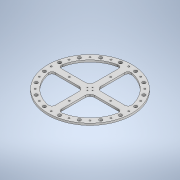
# Autodesk Inventor part: 24_Disco
Saved by Autodesk Inventor 2020.2 (Build 242310000, 310)
## iProperties
Created: 2019-11-29
Part Number: 24_Disco
Material: Generico
Document SubType Name: Modeling
Designer: socci
Density: 1 g/cm^3
Appearance: Default
Author: socci
Autodesk Inventor part; units mm, degrees
ref_plane "YZ Plane" through (0, 0, 0) normal (1, 0, 0) x (0, 1, 0)
ref_plane "XZ Plane" through (0, 0, 0) normal (0, 1, 0) x (-1, 0, 0)
ref_plane "XY Plane" through (0, 0, 0) normal (0, 0, 1) x (1, 0, 0)
sketch "Schizzo1" plane through (0, 0, 0) normal (0, 1, 0) x (-1, 0, 0)
  circle A0 centre (0, 0) radius 130
  line L0 (0, 130) -> (0, -130)
  line L1 (130, 0) -> (-130, 0)
  line L2 (10, 97.9796) -> (10, 23.6854)
  line L3 (97.9796, 10) -> (23.6854, 10)
  arc A1 (16.045, 13.5484) -> (13.5484, 16.045) centre (0, 0) ccw
  arc A2 (107.7775, 22) -> (22, 107.7775) centre (0, 0) ccw
  arc A3 (22, 107.7775) -> (10, 97.9796) centre (20, 97.9796) ccw
  arc A4 (10, 23.6854) -> (13.5484, 16.045) centre (20, 23.6854) ccw
  arc A5 (16.045, 13.5484) -> (23.6854, 10) centre (23.6854, 20) ccw
  arc A6 (97.9796, 10) -> (107.7775, 22) centre (97.9796, 20) ccw
  arc A7 (-13.5484, 16.045) -> (-10, 23.6854) centre (-20, 23.6854) ccw
  arc A8 (-13.5484, 16.045) -> (-16.045, 13.5484) centre (0, 0) ccw
  arc A9 (-23.6854, 10) -> (-16.045, 13.5484) centre (-23.6854, 20) ccw
  line L4 (-10, 97.9796) -> (-10, 23.6854)
  line L5 (-97.9796, 10) -> (-23.6854, 10)
  arc A10 (-107.7775, 22) -> (-97.9796, 10) centre (-97.9796, 20) ccw
  arc A11 (-22, 107.7775) -> (-107.7775, 22) centre (0, 0) ccw
  arc A12 (-10, 97.9796) -> (-22, 107.7775) centre (-20, 97.9796) ccw
  arc A13 (-16.045, -13.5484) -> (-23.6854, -10) centre (-23.6854, -20) ccw
  arc A14 (-16.045, -13.5484) -> (-13.5484, -16.045) centre (0, 0) ccw
  arc A15 (-10, -23.6854) -> (-13.5484, -16.045) centre (-20, -23.6854) ccw
  line L6 (-97.9796, -10) -> (-23.6854, -10)
  line L7 (-10, -97.9796) -> (-10, -23.6854)
  arc A16 (-22, -107.7775) -> (-10, -97.9796) centre (-20, -97.9796) ccw
  arc A17 (-107.7775, -22) -> (-22, -107.7775) centre (0, 0) ccw
  arc A18 (-97.9796, -10) -> (-107.7775, -22) centre (-97.9796, -20) ccw
  arc A19 (13.5484, -16.045) -> (10, -23.6854) centre (20, -23.6854) ccw
  arc A20 (13.5484, -16.045) -> (16.045, -13.5484) centre (0, 0) ccw
  arc A21 (23.6854, -10) -> (16.045, -13.5484) centre (23.6854, -20) ccw
  line L8 (10, -97.9796) -> (10, -23.6854)
  line L9 (97.9796, -10) -> (23.6854, -10)
  arc A22 (107.7775, -22) -> (97.9796, -10) centre (97.9796, -20) ccw
  arc A23 (22, -107.7775) -> (107.7775, -22) centre (0, 0) ccw
  arc A24 (10, -97.9796) -> (22, -107.7775) centre (20, -97.9796) ccw
  point P0 (18.4662, 10)
  point P1 (10, 18.4662)
  point P2 (109.5445, 10)
  point P3 (10, 109.5445)
  point P4 (-10, 18.4662)
  point P5 (-18.4662, 10)
  point P6 (-10, 109.5445)
  point P7 (-109.5445, 10)
  point P8 (-18.4662, -10)
  point P9 (-10, -18.4662)
  point P10 (-109.5445, -10)
  point P11 (-10, -109.5445)
  point P12 (10, -18.4662)
  point P13 (18.4662, -10)
  point P14 (10, -109.5445)
  point P15 (109.5445, -10)
  dimension "d0" = 260
  dimension "d2" = 10
  dimension "d5" = 10
  dimension "d7" = 10
  dimension "d10" = 360
  constraints: 68 point on circle, 25 centre point, 20 end point, 16 point on line, 8 tangent, 7 coincident, 3 equal radius, 2 parallel, 1 vertical, 107 other
  measures "d0" diameter of A0
  measures "d2" distance between parallel lines of L0 L2
  measures "d5" distance between parallel lines of L1 L3
  measures "d7" radius of A3
extrude "Estrusione1" add sketch "Schizzo1" along normal blind 6
sketch "Schizzo2" plane through (0, 6, 0) normal (0, 1, 0) x (1, 0, 0)
  line L0 (0, 0) -> (0, -8)
  line L1 (0, 0) -> (8, 0) construction
  point P0 (8, 0)
  point P1 (0, 8)
  point P2 (-8, 0)
  dimension "d14" = 8
  dimension "d15" = 90
  dimension "d18" = 360
  constraints: 4 end point, 1 coincident, 1 horizontal, 1 perpendicular, 1 vertical, 5 other
  measures "d14" distance of L0.start L0.end
  measures "d15" angle of L0 L1
hole "Foro1" at (0, 6, 8) at (0, 6, -8) at (8, 6, 0) at (-8, 6, 0) direction (0, -1, 0) diameter 3 end through all
sketch "Schizzo3" plane through (0, 6, 0) normal (0, 1, 0) x (1, 0, 0)
  line L0 (0, -110) -> (0, -130)
  circle A0 centre (0, 0) radius 130 projected
  line L1 (42.0952, -101.6267) -> (49.7488, -120.1043)
  line L2 (77.7817, -77.7817) -> (91.9239, -91.9239)
  line L3 (101.6267, -42.0952) -> (120.1043, -49.7488)
  line L4 (110, 0) -> (130, 0)
  line L5 (101.6267, 42.0952) -> (120.1043, 49.7488)
  line L6 (77.7817, 77.7817) -> (91.9239, 91.9239)
  line L7 (42.0952, 101.6267) -> (49.7488, 120.1043)
  line L8 (0, 110) -> (0, 130)
  line L9 (-42.0952, 101.6267) -> (-49.7488, 120.1043)
  line L10 (-77.7817, 77.7817) -> (-91.9239, 91.9239)
  line L11 (-101.6267, 42.0952) -> (-120.1043, 49.7488)
  line L12 (-110, 0) -> (-130, 0)
  line L13 (-101.6267, -42.0952) -> (-120.1043, -49.7488)
  line L14 (-77.7817, -77.7817) -> (-91.9239, -91.9239)
  line L15 (-42.0952, -101.6267) -> (-49.7488, -120.1043)
  circle A1 centre (0, -8) radius 1.5 projected
  line L16 (0, -8) -> (0, -120)
  point P0 (45.922, -110.8655)
  point P1 (84.8528, -84.8528)
  point P2 (110.8655, -45.922)
  point P3 (120, 0)
  point P4 (110.8655, 45.922)
  point P5 (84.8528, 84.8528)
  point P6 (45.922, 110.8655)
  point P7 (0, 120)
  point P8 (-45.922, 110.8655)
  point P9 (-84.8528, 84.8528)
  point P10 (-110.8655, 45.922)
  point P11 (-120, 0)
  point P12 (-110.8655, -45.922)
  point P13 (-84.8528, -84.8528)
  point P14 (-45.922, -110.8655)
  point P15 (0, -64)
  point P16 (64, 0)
  point P17 (0, 64)
  point P18 (-64, 0)
  dimension "d29" = 360
  dimension "d33" = 360
  constraints: 34 end point, 4 coincident, 2 midpoint, 2 vertical, 1 vertical alignment, 87 other
hole "Foro2" at (0, 6, 120) at (45.922, 6, 110.8655) at (84.8528, 6, 84.8528) at (110.8655, 6, 45.922) at (120, 6, 0) at (110.8655, 6, -45.922) at (84.8528, 6, -84.8528) at (45.922, 6, -110.8655) at (0, 6, -120) at (-45.922, 6, -110.8655) at (-84.8528, 6, -84.8528) at (-110.8655, 6, -45.922) at (-120, 6, 0) at (-110.8655, 6, 45.922) at (-84.8528, 6, 84.8528) at (-45.922, 6, 110.8655) at (0, 6, 64) at (64, 6, 0) at (0, 6, -64) at (-64, 6, 0) direction (0, -1, 0) diameter 5 end through all
sketch "Schizzo4" plane through (0, 6, 0) normal (0, 1, 0) x (1, 0, 0)
  circle A0 centre (0, -120) radius 2.5 projected
  circle A1 centre (45.922, -110.8655) radius 2.5 projected
  arc A2 (0, -120) -> (45.922, -110.8655) centre (0, 0) ccw
  point P0 (23.4108, -117.6942)
  point P1 (66.6684, -99.7764)
  point P2 (99.7764, -66.6684)
  point P3 (117.6942, -23.4108)
  point P4 (117.6942, 23.4108)
  point P5 (99.7764, 66.6684)
  point P6 (66.6684, 99.7764)
  point P7 (23.4108, 117.6942)
  point P8 (-23.4108, 117.6942)
  point P9 (-66.6684, 99.7764)
  point P10 (-99.7764, 66.6684)
  point P11 (-117.6942, 23.4108)
  point P12 (-117.6942, -23.4108)
  point P13 (-99.7764, -66.6684)
  point P14 (-66.6684, -99.7764)
  point P15 (-23.4108, -117.6942)
  dimension "d44" = 360
  constraints: 3 point on circle, 1 centre point, 1 coincident, 17 other
hole "Foro3" at (23.4108, 6, 117.6942) at (66.6684, 6, 99.7764) at (99.7764, 6, 66.6684) at (117.6942, 6, 23.4108) at (117.6942, 6, -23.4108) at (99.7764, 6, -66.6684) at (66.6684, 6, -99.7764) at (23.4108, 6, -117.6942) at (-23.4108, 6, -117.6942) at (-66.6684, 6, -99.7764) at (-99.7764, 6, -66.6684) at (-117.6942, 6, -23.4108) at (-117.6942, 6, 23.4108) at (-99.7764, 6, 66.6684) at (-66.6684, 6, 99.7764) at (-23.4108, 6, 117.6942) direction (0, -1, 0) diameter 10 end through all
